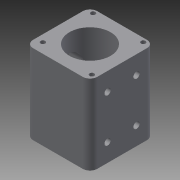
# Autodesk Inventor part: nema23_motor_mount
Saved by Autodesk Inventor 2014 (Build 180170000, 170)
## iProperties
Created: 2014-08-14
Part Number: nema23_motor_mount
Material: Generic
Document SubType Name: Modeling
Designer: Matthew
Density: 1 g/cm^3
Appearance: Default
Mass: 131.767 g
Surface Area: 307.867 cm^2
Volume: 131.767 cm^3
Author: Matthew
Autodesk Inventor part; units mm, degrees
ref_plane "YZ Plane" through (0, 0, 0) normal (1, 0, 0) x (0, 1, 0)
ref_plane "XZ Plane" through (0, 0, 0) normal (0, 1, 0) x (-1, 0, 0)
ref_plane "XY Plane" through (0, 0, 0) normal (0, 0, 1) x (1, 0, 0)
sketch "Sketch1" plane through (0, 0, 0) normal (0, 1, 0) x (-1, 0, 0)
  line L0 (28.1305, 28.1305) -> (-28.1305, 28.1305)
  line L1 (-28.1305, 28.1305) -> (-28.1305, -28.1305)
  line L2 (-28.1305, -28.1305) -> (28.1305, -28.1305)
  line L3 (28.1305, -28.1305) -> (28.1305, 28.1305)
  line L4 (28.1305, 28.1305) -> (-28.1305, -28.1305) construction
  line L5 (-28.1305, 28.1305) -> (28.1305, -28.1305) construction
  point P0 (0, 0)
  dimension "d0" = 56.261
  dimension "d1" = 56.261
  constraints: 12 end point, 2 midpoint, 2 parallel, 1 horizontal, 1 perpendicular
  measures "d0" distance of L0.end L1.end
  measures "d1" distance of L1.end L2.end
extrude "Extrusion1" add sketch "Sketch1" along normal blind 69.85
sketch "Sketch2" plane through (0, 69.85, 0) normal (0, 1, 0) x (1, 0, 0)
  circle A0 centre (0, 0) radius 18
  point P0 (-22, 24.7091)
  point P1 (22, 24.7091)
  point P2 (24.0589, -22.4333)
  point P3 (-22, -19.2909)
  dimension "d4" = 44
  dimension "d5" = 44
  dimension "d6" = 22
  dimension "d7" = 36
  constraints: 1 centre point, 1 coincident
  measures "d4" distance of point (-22, -19.291) point (-22, 24.709)
  measures "d5" distance of point (22, 24.709) point (-22, 24.709)
  measures "d6" horizontal distance of point (0, 0) point (-22, 24.709)
  measures "d7" diameter of A0
hole "Hole1" at (-22, 69.85, -24.7091) at (22, 69.85, -24.7091) at (24.0589, 69.85, 22.4333) at (-22, 69.85, 19.2909) direction (0, -1, 0) diameter 4 depth 25.4 tip angle 118
sketch "Sketch3" plane through (0, 69.85, 0) normal (0, 1, 0) x (1, 0, 0)
  circle A0 centre (0, 0) radius 18
  dimension "d15" = 36
  constraints: 1 centre point, 1 coincident
  measures "d15" diameter of A0
extrude "Extrusion2" cut sketch "Sketch3" against normal blind 254
sketch "Sketch4" plane through (0, 0, 0) normal (0, -1, 0) x (1, 0, 0)
  circle A0 centre (0, 0) radius 18 projected
  point P0 (-23.3446, 23.5712)
  point P1 (23.7978, 23.5712)
  point P2 (23.7978, -23.5712)
  point P3 (-23.3446, -23.5712)
  dimension "d18" = 47.1424
  dimension "d19" = 47.1424
  dimension "d20" = 23.5712
  constraints: 2 horizontal alignment, 2 vertical alignment
  measures "d18" distance of point (23.798, 23.571) point (-23.345, 23.571)
  measures "d19" distance of point (-23.345, 23.571) point (-23.345, -23.571)
  measures "d20" vertical distance of A0.centre point (23.798, -23.571)
hole "Hole2" at (-23.3446, 0, 23.5712) at (23.7978, 0, 23.5712) at (23.7978, 0, -23.5712) at (-23.3446, 0, -23.5712) direction (0, 1, 0) diameter 5 depth 25.4 tip angle 118
sketch "Sketch5" plane through (0, 0, 0) normal (0, -1, 0) x (1, 0, 0)
  circle A0 centre (0, 0) radius 18 projected
  circle A1 centre (0, 0) radius 19.0754
  dimension "d28" = 38.1508
  constraints: 1 centre point, 1 coincident
  measures "d28" diameter of A1
extrude "Extrusion3" cut sketch "Sketch5" against normal blind 34.925
fillet "Fillet1" radius 6.35 1 edges at (28.1305, 34.925, 28.1305)
fillet "Fillet2" radius 6.35 1 edges at (-28.1305, 34.925, 28.1305)
fillet "Fillet3" radius 6.35 1 edges at (28.1305, 34.925, -28.1305)
fillet "Fillet4" radius 6.35 1 edges at (-28.1305, 34.925, -28.1305)
sketch "Sketch6" plane through (-28.1305, 0, 21.7805) normal (-1, 0, 0) x (0, 0, 1)
  line L0 (-49.911, 0) -> (0, 0) projected
  line L1 (0, 69.85) -> (0, 0) projected
  line L2 (-31.3055, 25.4) -> (-12.2555, 25.4) construction
  line L3 (-12.2555, 25.4) -> (-12.2555, 44.45)
  line L4 (-12.2555, 44.45) -> (-31.3055, 44.45) construction
  line L5 (-31.3055, 44.45) -> (-31.3055, 25.4)
  line L6 (-31.3055, 25.4) -> (-12.2555, 44.45) construction
  line L7 (-12.2555, 25.4) -> (-31.3055, 44.45) construction
  arc A0 (-12.2555, 44.45) -> (-31.3055, 44.45) centre (-21.7805, 44.45) ccw
  arc A1 (-31.3055, 25.4) -> (-12.2555, 25.4) centre (-21.7805, 25.4) ccw
  point P0 (-43.561, 0)
  point P1 (-21.7805, 0)
  point P2 (-21.7805, 34.925)
  point P3 (-21.7805, 34.925)
  point P4 (-21.7805, 0)
  point P5 (0, 34.925)
  point P6 (-21.7805, 53.975)
  point P7 (-21.7805, 15.875)
  dimension "d35" = 19.05
  dimension "d36" = 19.05
  constraints: 12 end point, 6 midpoint, 6 point on circle, 2 centre point, 2 parallel, 1 horizontal, 1 horizontal alignment, 1 perpendicular, 1 point on line, 1 vertical alignment
  measures "d35" distance of L4.end L3.end
  measures "d36" distance of L2.end L3.end
extrude "Extrusion4" cut sketch "Sketch6" against normal blind 25.4
sketch "Sketch7" plane through (28.1305, 0, 21.7805) normal (1, 0, 0) x (0, 0, -1)
  line L0 (0, 0) -> (0, 69.85) projected
  line L1 (0, 0) -> (49.911, 0) projected
  line L2 (9.0805, 15.875) -> (34.4805, 15.875) construction
  line L3 (34.4805, 15.875) -> (34.4805, 53.975) construction
  line L4 (34.4805, 53.975) -> (9.0805, 53.975) construction
  line L5 (9.0805, 53.975) -> (9.0805, 15.875) construction
  line L6 (9.0805, 15.875) -> (34.4805, 53.975) construction
  line L7 (34.4805, 15.875) -> (9.0805, 53.975) construction
  line L8 (0, 69.85) -> (49.911, 69.85) projected
  point P0 (43.561, 0)
  point P1 (21.7805, 0)
  point P2 (21.7805, 34.925)
  point P3 (21.7805, 0)
  point P4 (0, 34.925)
  point P5 (43.561, 69.85)
  dimension "d39" = 25.4
  dimension "d40" = 38.1
  dimension "d48" = 15.875
  constraints: 12 end point, 4 coincident, 3 midpoint, 2 parallel, 1 horizontal, 1 horizontal alignment, 1 perpendicular, 1 point on line, 1 vertical alignment
  measures "d39" distance of L4.end L3.end
  measures "d40" distance of L2.end L3.end
  measures "d48" distance between parallel lines of L4 L8
hole "Hole3" at (28.1305, 53.975, 12.7) at (28.1305, 53.975, -12.7) at (28.1305, 15.875, -12.7) at (28.1305, 15.875, 12.7) direction (-1, 0, 0) diameter 5.5 depth 25.4 tip angle 118
equation "\"d5\" = d4"
equation "\"d6\" = 0.5 * d4"
equation "\"d19\" = d18"
equation "\"d20\" = 0.5 * d18"
body "Solid1"
